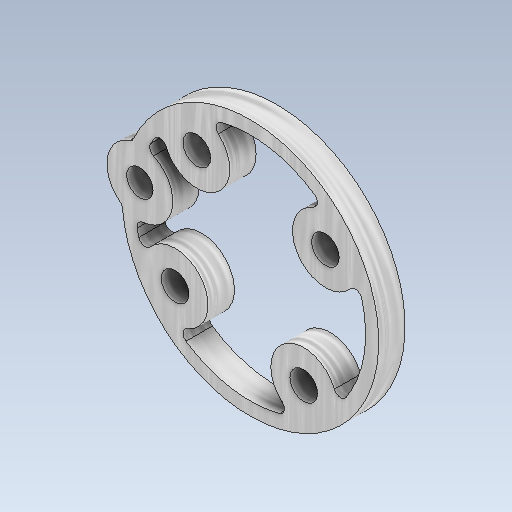
# Autodesk Inventor part: 横回転首振り駆動
Saved by Autodesk Inventor 2020 (Build 240168000, 168)
## iProperties
Created: 2020-02-26
Part Number: 横回転首振り駆動
Material: アルミニウム 7075
Document SubType Name: Modeling
Designer: tanjihayato
Density: 2.81 g/cm^3
Appearance: サテン - ブラシ仕上げ 重厚
Mass: 5.75795 g
Surface Area: 23.9798 cm^2
Volume: 2.04909 cm^3
Author: tanjihayato
Autodesk Inventor part; units mm, degrees
ref_plane "YZ Plane" through (0, 0, 0) normal (1, 0, 0) x (0, 1, 0)
ref_plane "XZ Plane" through (0, 0, 0) normal (0, 1, 0) x (-1, 0, 0)
ref_plane "XY Plane" through (0, 0, 0) normal (0, 0, 1) x (1, 0, 0)
sketch "スケッチ1" plane through (0, 0, 0) normal (0, 0, 1) x (1, 0, 0)
  circle A0 centre (-11.4931, -19.1593) radius 14 construction
  circle A1 centre (16.245, -15.3385) radius 14 construction
  line L0 (-170.915, -81.4118) -> (490.0044, -81.4118)
  line L1 (-197.2268, -33.1593) -> (179.6604, -33.1593) construction
  line L2 (-178.6504, 68.5882) -> (447.0756, 68.5882) construction
  circle A2 centre (-11.4931, -19.1593) radius 14 construction
  circle A3 centre (-21.8854, 6.8407) radius 14 construction
  circle A4 centre (-0.5211, 0.3031) radius 20.05 construction
  circle A5 centre (-0.5211, 0.3031) radius 22.3421 construction
  circle A6 centre (0, 0) radius 22.3421 construction
  circle A7 centre (-0.5211, 0.3031) radius 5.05 construction
  circle A8 centre (19.689, 29.6103) radius 30.55 construction
  circle A9 centre (19.689, 29.6103) radius 10.1 construction
  circle A10 centre (39.672, 58.5882) radius 25.1 construction
  line L3 (-0.5211, 0.3031) -> (39.672, 58.5882) construction
  circle A11 centre (39.672, 58.5882) radius 27.1 construction
  circle A12 centre (19.689, 29.6103) radius 31.55 construction
  circle A13 centre (19.689, 29.6103) radius 12.1 construction
  circle A14 centre (-0.5211, 0.3031) radius 20.55 construction
  circle A15 centre (-0.5211, 0.3031) radius 6.05 construction
  circle A16 centre (36.8436, 61.4166) radius 4 construction
  circle A17 centre (36.8436, 61.4166) radius 2
  line L4 (36.8436, 61.4166) -> (39.672, 58.5882)
  line L5 (39.672, 58.5882) -> (22.909, 61.4166) construction
  circle A18 centre (22.909, 61.4166) radius 2
  circle A19 centre (22.909, 61.4166) radius 5
  line L6 (28.2635, 50.4737) -> (31.5576, 69.9968) construction
  line L7 (31.5576, 69.9968) -> (51.0806, 66.7027) construction
  line L8 (51.0806, 66.7027) -> (47.7865, 47.1796) construction
  line L9 (47.7865, 47.1796) -> (28.2635, 50.4737) construction
  circle A20 centre (39.672, 58.5882) radius 9
  circle A21 centre (28.2635, 50.4737) radius 2.5
  circle A22 centre (47.7865, 47.1796) radius 2.5
  circle A23 centre (51.0806, 66.7027) radius 2.5
  circle A24 centre (31.5576, 69.9968) radius 2.5
  circle A25 centre (28.2635, 50.4737) radius 5
  line L10 (22.909, 61.4166) -> (36.8436, 61.4166) construction
  line L11 (-26.0808, 51.4166) -> (-426.0808, 51.4166)
  line L12 (-26.0808, 24.4166) -> (23.9192, 24.4166)
  circle A26 centre (39.672, 58.5882) radius 17.5
  circle A27 centre (47.7865, 47.1796) radius 2.1
  circle A28 centre (28.2635, 50.4737) radius 2.1
  circle A29 centre (31.5576, 69.9968) radius 2.1
  circle A30 centre (51.0806, 66.7027) radius 2.1
  circle A31 centre (47.7865, 47.1796) radius 5
  circle A32 centre (31.5576, 69.9968) radius 5
  circle A33 centre (51.0806, 66.7027) radius 5
  circle A34 centre (39.672, 58.5882) radius 19.5
  circle A35 centre (39.672, 58.5882) radius 20.5
  line L13 (20.7504, 89.6882) -> (53.4998, 89.6882)
  line L14 (53.4998, 89.6882) -> (73.6516, 68.9857)
  line L15 (20.7504, 89.6882) -> (-13.977, 39.0272)
  circle A36 centre (-59.2702, 32.0272) radius 5.025 construction
  circle A37 centre (-59.2702, 32.0272) radius 4
  arc A38 (-59.2702, 39.0272) -> (-62.5897, 25.8643) centre (-59.2702, 32.0272) ccw
  line L16 (-59.2702, 39.0272) -> (-13.977, 39.0272)
  line L17 (-62.5897, 25.8643) -> (-36.5547, 11.8407)
  line L18 (-36.5547, 11.8407) -> (-36.5547, -33.1593)
  arc A39 (74.5655, 64.0796) -> (73.6516, 68.9857) centre (70.4271, 65.8469) ccw
  circle A40 centre (8.5193, 63.8863) radius 4.5 construction
  arc A41 (59.4085, 28.8085) -> (59.8353, 29.5856) centre (55.6969, 31.3528) ccw
  circle A42 centre (23.6647, -6.2198) radius 4.5
  circle A43 centre (-16.0241, 34.5272) radius 4.5 construction
  line L19 (59.8353, 29.5856) -> (74.5655, 64.0796)
  line L20 (32.172, 89.6882) -> (32.172, 92.6882)
  line L21 (32.172, 92.6882) -> (47.172, 92.6882)
  line L22 (47.172, 92.6882) -> (47.172, 89.6882)
  line L23 (35.172, 89.6882) -> (35.172, 86.6882)
  line L24 (35.172, 86.6882) -> (44.172, 86.6882)
  line L25 (44.172, 86.6882) -> (44.172, 89.6882)
  circle A44 centre (70.4271, 65.8469) radius 1.5
  circle A45 centre (55.6969, 31.3528) radius 1.5
  circle A46 centre (23.6647, -6.2198) radius 1.5
  circle A47 centre (-16.0241, 34.5272) radius 1.5
  circle A48 centre (8.5193, 63.8863) radius 1.5
  circle A49 centre (-10.0662, 20.4166) radius 4 construction
  circle A50 centre (-10.0662, 20.4166) radius 2
  line L26 (1.9305, -36.1593) -> (16.9305, -36.1593)
  line L27 (16.9305, -36.1593) -> (16.9305, -33.1593)
  line L28 (1.9305, -33.1593) -> (1.9305, -36.1593)
  arc A51 (1.9305, -33.1593) -> (-0.1695, -33.1593) centre (0.8805, -33.1593) ccw
  line L29 (13.9305, -30.1593) -> (13.9305, -33.1593)
  arc A52 (13.9305, -30.1593) -> (11.8305, -30.1593) centre (12.8805, -30.1593) ccw
  line L30 (7.0305, -30.1593) -> (11.8305, -30.1593)
  arc A53 (7.0305, -30.1593) -> (4.9305, -30.1593) centre (5.9805, -30.1593) ccw
  line L31 (4.9305, -33.1593) -> (4.9305, -30.1593)
  arc A54 (4.9305, -33.1593) -> (7.0305, -33.1593) centre (5.9805, -33.1593) ccw
  arc A55 (11.8305, -33.1593) -> (13.9305, -33.1593) centre (12.8805, -33.1593) ccw
  line L32 (-36.5547, -36.1593) -> (-21.5547, -36.1593)
  line L33 (-21.5547, -36.1593) -> (-21.5547, -33.1593)
  arc A56 (-19.4547, -33.1593) -> (-21.5547, -33.1593) centre (-20.5047, -33.1593) ccw
  line L34 (-36.5547, -33.1593) -> (-36.5547, -36.1593)
  arc A57 (-33.5547, -33.1593) -> (-31.4547, -33.1593) centre (-32.5047, -33.1593) ccw
  line L35 (-33.5547, -33.1593) -> (-33.5547, -30.1593)
  arc A58 (-31.4547, -30.1593) -> (-33.5547, -30.1593) centre (-32.5047, -30.1593) ccw
  line L36 (-31.4547, -30.1593) -> (-26.6547, -30.1593)
  arc A59 (-24.5547, -30.1593) -> (-26.6547, -30.1593) centre (-25.6047, -30.1593) ccw
  line L37 (-24.5547, -30.1593) -> (-24.5547, -33.1593)
  arc A60 (-26.6547, -33.1593) -> (-24.5547, -33.1593) centre (-25.6047, -33.1593) ccw
  line L38 (59.4085, 28.8085) -> (16.9305, -33.1593)
  circle A61 centre (-21.8854, 6.8407) radius 5
  circle A62 centre (-11.4931, -19.1593) radius 5
  line L39 (-31.4547, -33.1593) -> (-26.6547, -33.1593)
  line L40 (-19.4547, -33.1593) -> (-0.1695, -33.1593)
  line L41 (7.0305, -33.1593) -> (11.8305, -33.1593)
  line L42 (0.4485, -25.8914) -> (-27.1419, -10.3373) construction
  line L43 (-27.1419, -10.3373) -> (-17.3768, 21.5744) construction
  circle A63 centre (-21.8854, 6.8407) radius 8
  circle A64 centre (-11.4931, -19.1593) radius 8
  circle A65 centre (-19.5445, 14.4905) radius 1.3
  circle A66 centre (-24.2262, -0.8092) radius 1.3
  circle A67 centre (-18.4619, -15.2306) radius 1.3
  circle A68 centre (-4.5242, -23.088) radius 1.3
  circle A69 centre (-0.5211, 0.3031) radius 4.5
  circle A70 centre (19.689, 29.6103) radius 6
  arc A71 (87.3323, 12.0445) -> (87.1264, 18.8999) centre (85.1711, 15.4104) ccw
  line L44 (16.9305, -33.1593) -> (87.3323, 12.0445)
  line L45 (87.1264, 18.8999) -> (61.4227, 33.3027)
  circle A72 centre (85.1711, 15.4104) radius 2
  point P0 (21.7537, 66.2813)
  point P1 (20.2215, 57.2003)
  point P2 (33.0249, 74.7766)
  point P3 (51.2629, 71.6993)
  point P4 (55.8605, 65.2354)
  point P5 (52.7832, 46.9973)
  point P6 (46.3192, 42.3998)
  point P7 (28.0812, 45.4771)
  point P8 (23.4836, 51.941)
  point P9 (22.3027, 56.4535)
  point P10 (23.9648, 66.3039)
  point P11 (26.5609, 70.1791)
  dimension "d0" = 150
  dimension "d1" = 28
  dimension "d2" = 28
  dimension "d3" = 40.1
  dimension "d4" = 10.1
  dimension "d5" = 61.1
  dimension "d6" = 20.2
  dimension "d7" = 50.2
  dimension "d8" = 10
  dimension "d9" = 2
  dimension "d10" = 1
  dimension "d11" = 2
  dimension "d12" = 0.5
  dimension "d13" = 1
  dimension "d14" = 40
  dimension "d15" = 8
  dimension "d16" = 4
  dimension "d17" = 4
  dimension "d18" = 45
  dimension "d19" = 17
  dimension "d20" = 4
  dimension "d21" = 3
  dimension "d22" = 1
  dimension "d23" = 5
  dimension "d24" = 5
  dimension "d25" = 5
  dimension "d26" = 5
  dimension "d27" = 10
  dimension "d28" = 400
  dimension "d29" = 10
  dimension "d30" = 50
  dimension "d31" = 50
  dimension "d32" = 27
  dimension "d33" = 27
  dimension "d34" = 35
  dimension "d35" = 4.2
  dimension "d36" = 4.2
  dimension "d37" = 4.2
  dimension "d38" = 4.2
  dimension "d39" = 10
  dimension "d40" = 10
  dimension "d41" = 10
  dimension "d42" = 2
  dimension "d43" = 1
  dimension "d44" = 8
  dimension "d45" = 3
  dimension "d46" = 4
  dimension "d47" = 9
  dimension "d48" = 9
  dimension "d49" = 9
  dimension "d50" = 9
  dimension "d51" = 9
  dimension "d52" = 3
  dimension "d53" = 15
  dimension "d54" = 3
  dimension "d55" = 9
  dimension "d56" = 3
  dimension "d57" = 7.5
  dimension "d58" = 3
  dimension "d59" = 3
  dimension "d60" = 3
  dimension "d61" = 3
  dimension "d62" = 3
  dimension "d63" = 8
  constraints: 90 end point, 71 centre point, 34 point on circle, 32 coincident, 23 tangent, 12 point on line, 7 perpendicular, 6 horizontal, 3 parallel, 1 collinear, 1 equal radius, 1 vertical, 22 other
  measures "d0" distance between parallel lines of L0 L2
  measures "d1" diameter of A2
  measures "d2" diameter of A3
  measures "d3" diameter of A4
  measures "d4" diameter of A7
  measures "d5" diameter of A8
  measures "d6" diameter of A9
  measures "d7" diameter of A10
  measures "d8" distance from line of L2 L3.end
  measures "d10" radial gap between concentric circles of A8 A12
  measures "d11" radial gap between concentric circles of A9 A13
  measures "d12" radial gap between concentric circles of A4 A14
  measures "d13" radial gap between concentric circles of A7 A15
  measures "d15" diameter of A16
  measures "d16" diameter of A17
  measures "d17" distance of A16.centre L3.end
  measures "d18" angle of L0 L4
  measures "d19" distance of L3.end L5.end
  measures "d20" diameter of A18
  measures "d21" radial gap between concentric circles of A18 A19
  measures "d23" diameter of A21
  measures "d24" diameter of A22
  measures "d25" diameter of A23
  measures "d26" diameter of A24
  measures "d27" diameter of A25
  measures "d28" distance of L11.start L11.end
  measures "d29" distance between parallel lines of L10 L11
  measures "d30" distance of L5.end L11.start
  measures "d31" distance of L12.start L12.end
  measures "d32" distance between parallel lines of L12 L11
  measures "d33" distance of L11.start L12.start
  measures "d34" diameter of A26
  measures "d35" diameter of A27
  measures "d36" diameter of A28
  measures "d37" diameter of A29
  measures "d38" diameter of A30
  measures "d39" diameter of A31
  measures "d40" diameter of A32
  measures "d41" diameter of A33
  measures "d42" radial gap between concentric circles of A26 A34
  measures "d43" radial gap between concentric circles of A34 A35
  measures "d44" diameter of A37
  measures "d45" radial gap between concentric circles of A37 A38
  measures "d47" diameter of A39
  measures "d48" diameter of A40
  measures "d49" diameter of A41
  measures "d50" diameter of A42
  measures "d51" diameter of A43
  measures "d52" distance of L20.start L20.end
  measures "d53" distance of L20.end L21.end
  measures "d54" distance of L23.start L23.end
  measures "d55" distance of L23.end L24.end
  measures "d56" distance between parallel lines of L22 L25
  measures "d57" distance from line of L3.end L20
  measures "d58" diameter of A44
  measures "d59" diameter of A45
  measures "d60" diameter of A46
  measures "d61" diameter of A47
  measures "d62" diameter of A48
  measures "d63" diameter of A49
extrude "押し出し1" add sketch "スケッチ1" along normal blind 4 contours A18 A26 A19 | A18 A26 A19 A34 | A19 A34 A26 A25 A31 A33 A32 | A34 A19 A35 | A32 A26 | A26 A32 | A26 A25 | A25 A26 | A35 A19 | A33 A26 | A26 A33 | A31 A26 | A26 A31 | A21 | A22 | A23 | A24 picked at (20.0967, 61.4489)
fillet "フィレット1" radius 1 12 edges at (21.7537, 66.2813, 2) (20.2215, 57.2003, 2) (26.5609, 70.1791, 2) (33.0249, 74.7766, 2) (23.9648, 66.3039, 2) (22.3027, 56.4535, 2) (23.4836, 51.941, 2) (28.0812, 45.4771, 2) (46.3192, 42.3998, 2) (52.7832, 46.9973, 2) (55.8605, 65.2354, 2) (51.2629, 71.6993, 2)
